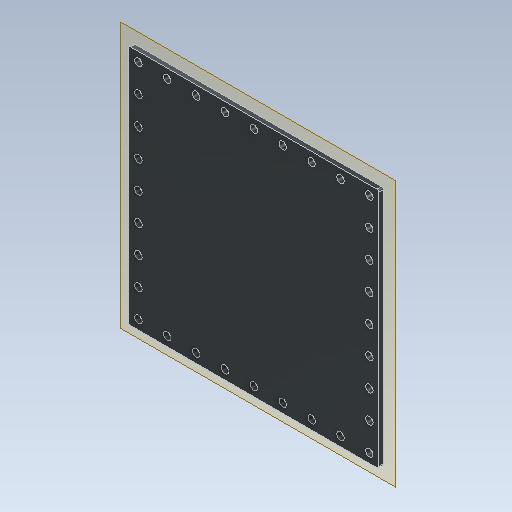
# Autodesk Inventor part: Крышка воды зад
Saved by Autodesk Inventor 2021 (Build 250183000, 183)
## iProperties
Created: 2020-11-22
Part Number: Крышка воды зад
Material: Чугун, серый
Document SubType Name: Modeling
Designer: Тимоха
Mass: 2445.26 g
Surface Area: 1460.94 cm^2
Volume: 341.994 cm^3
Density: 7.15 g/cm^3
Appearance: Чугун серый
Author: Тимоха
Autodesk Inventor part; units mm, degrees
ref_plane "YZ Plane" through (0, 0, 0) normal (1, 0, 0) x (0, 1, 0)
ref_plane "XZ Plane" through (0, 0, 0) normal (0, 1, 0) x (-1, 0, 0)
ref_plane "XY Plane" through (0, 0, 0) normal (0, 0, 1) x (1, 0, 0)
ref_plane "РабПлоскость1" through (0, 0, 0) normal (0, 0, 1) x (1, 0, 0)
sketch "Эскиз1" plane through (0, 0, 0) normal (0, 0, 1) x (1, 0, 0)
  line L0 (-132.636, -130) -> (132.636, -130) projected
  arc A0 (132.636, -130) -> (134.636, -128) centre (132.636, -128) ccw projected
  line L1 (134.636, -128) -> (134.636, 128) projected
  arc A1 (134.636, 128) -> (132.636, 130) centre (132.636, 128) ccw projected
  line L2 (132.636, 130) -> (-132.636, 130) projected
  arc A2 (-132.636, 130) -> (-134.636, 128) centre (-132.636, 128) ccw projected
  line L3 (-134.636, 128) -> (-134.636, -128) projected
  arc A3 (-134.636, -128) -> (-132.636, -130) centre (-132.636, -128) ccw projected
  circle A4 centre (124.636, 120) radius 4 projected
  circle A5 centre (62.436, 120) radius 4 projected
  circle A6 centre (0.236, 120) radius 4 projected
  circle A7 centre (-61.964, 120) radius 4 projected
  circle A8 centre (-124.164, 120) radius 4 projected
  circle A9 centre (-124.164, 90) radius 4 projected
  circle A10 centre (-124.164, 60) radius 4 projected
  circle A11 centre (-124.164, 30) radius 4 projected
  circle A12 centre (-124.164, 0) radius 4 projected
  circle A13 centre (-124.164, -30) radius 4 projected
  circle A14 centre (-124.164, -60) radius 4 projected
  circle A15 centre (-124.164, -90) radius 4 projected
  circle A16 centre (93.536, -120) radius 4 projected
  circle A17 centre (62.436, -120) radius 4 projected
  circle A18 centre (31.336, -120) radius 4 projected
  circle A19 centre (0.236, -120) radius 4 projected
  circle A20 centre (-30.864, -120) radius 4 projected
  circle A21 centre (-61.964, -120) radius 4 projected
  circle A22 centre (-93.064, -120) radius 4 projected
  circle A23 centre (-124.164, -120) radius 4 projected
  circle A24 centre (124.636, -120) radius 4 projected
  circle A25 centre (124.636, -90) radius 4 projected
  circle A26 centre (124.636, -60) radius 4 projected
  circle A27 centre (124.636, -30) radius 4 projected
  circle A28 centre (124.636, 0) radius 4 projected
  circle A29 centre (124.636, 30) radius 4 projected
  circle A30 centre (124.636, 60) radius 4 projected
  circle A31 centre (124.636, 90) radius 4 projected
  circle A32 centre (-93.064, 120) radius 4 projected
  circle A33 centre (-30.864, 120) radius 4 projected
  circle A34 centre (31.336, 120) radius 4 projected
  circle A35 centre (93.536, 120) radius 4 projected
  line L4 (-115.364, -110) -> (-115.364, 110) projected
  line L5 (-115.364, 110) -> (114.636, 110) projected
  line L6 (114.636, 110) -> (114.636, -110) projected
  line L7 (114.636, -110) -> (-115.364, -110) projected
  point P0 (0, 0)
extrude "Выдавливание1" add sketch "Эскиз1" along normal blind 5 contours A3 L3 A2 L2 A1 L1 A0 L0 | L4 L5 L6 L7
